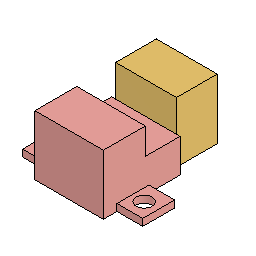
RoBo fan (Autodesk Fusion 360 archive; units mm, degrees)
design "male female connector"
Autodesk Fusion 360 part; units mm, degrees
sketch "Sketch1" plane through (0, 0, 0) normal (0, 0, 1) x (1, 0, 0) in component "male"
  line L0 (8.57, -9.6) -> (-8.57, -9.6)
  line L1 (-8.57, -9.6) -> (-8.57, 9.6)
  line L2 (-8.57, 9.6) -> (8.57, 9.6)
  line L3 (8.57, 9.6) -> (8.57, -9.6)
  line L4 (8.57, -9.6) -> (-8.57, 9.6) construction
  line L5 (-8.57, -9.6) -> (8.57, 9.6) construction
  line L6 (15.03, 1.8) -> (15.03, -6.2)
  line L7 (-15.03, -6.2) -> (-15.03, 1.8)
  line L8 (0, -6.2) -> (0, 0) construction
  circle A0 centre (-11.58, -2.4) radius 2
  circle A1 centre (11.58, -2.4) radius 2
  line L9 (-11.58, -2.4) -> (11.58, -2.4) construction
  line L10 (0, -2.4) -> (0, -6.2) construction
  line L11 (8.57, 0.9) -> (-8.57, 0.9)
  line L12 (-15.03, 1.8) -> (-8.57, 1.8)
  line L13 (8.57, 1.8) -> (15.03, 1.8)
  line L14 (15.03, -6.2) -> (8.57, -6.2)
  line L15 (-8.57, -6.2) -> (-15.03, -6.2)
  dimension "d1" = 17.14
  dimension "d2" = 19.2
  dimension "d4" = 8
  dimension "d5" = 7.8
  dimension "d6" = 4
  dimension "d7" = 23.16
  dimension "d8" = 3.8
  dimension "d9" = 6.46
  dimension "d14" = 8.7
  constraint horizontal L0
  constraint perpendicular L0 L1
  constraint parallel L0 L2
  constraint parallel L1 L3
  constraint coincident L4 L8.end
  constraint coincident L5 L8.end
  constraint coincident L8.end origin
  constraint horizontal L12
  constraint vertical L6
  constraint horizontal L14
  constraint vertical L7
  constraint vertical L8
  constraint coincident A0.centre L9.start
  constraint coincident A1.centre L9.end
  constraint horizontal L9
  constraint equal A0 A1
  constraint midpoint L9 L10.start
  constraint vertical L10
  constraint coincident L3 L11.start
  constraint coincident L1 L11.end
  constraint perpendicular L1 L11
  constraint coincident L3 L13.start
  constraint collinear L12 L13
  constraint coincident L1 L12.end
  constraint collinear L14 L15
  constraint coincident L3 L14.end
  constraint coincident L1 L15.start
  constraint equal L14 L15
  measures "d1" distance of L1.end L2.end
  measures "d2" distance of L0.end L1.end
  measures "d4" distance of L7.end L7.start
  measures "d5" distance of L1.end L12
  measures "d6" diameter of A0
  measures "d7" distance of A0.centre A1.centre
  measures "d8" distance of L9 L14
  measures "d9" distance of L1 L7.end
  measures "d14" distance of L2 L11
extrude "Extrude1" add sketch "Sketch1" along normal blind 1.74 contours L3 L6 L13 L14 | L1 L7 L12 L15 makes body 1 at (-11.7765, 1.0648, 0) makes body 2 at (11.7765, 1.0648, 0) in component "male"
extrude "Extrude3" add sketch "Sketch1" along normal blind 8.4 contours L1 L2 L3 L11 bodies 1 2 in component "male"
extrude "Extrude4" add sketch "Sketch1" along normal blind 15 contours L0 L1 L3 L11 bodies 1 in component "male"
sketch "Sketch1 (2)" plane through (0, 0, 0) normal (0, 0, 1) x (1, 0, 0) in component "female"
  line L0 (9.3617, 28.1045) -> (-5.8783, 28.1045)
  line L1 (-5.8783, 28.1045) -> (-5.8783, 47.0045)
  line L2 (-5.8783, 47.0045) -> (9.3617, 47.0045)
  line L3 (9.3617, 47.0045) -> (9.3617, 28.1045)
  line L4 (9.3617, 36.8045) -> (-5.8783, 36.8045)
  dimension "d19" = 15.24
  dimension "d20" = 18.9
  dimension "d21" = 8.7
  constraint horizontal L0
  constraint vertical L1
  constraint horizontal L2
  constraint vertical L3
  constraint coincident L3 L4.start
  constraint coincident L1 L4.end
  constraint perpendicular L1 L4
  measures "d19" distance of L0.start L0.end
  measures "d20" distance of L0.start L2.end
  measures "d21" distance of L0 L4
extrude "Extrude1'" add sketch "Sketch1 (2)" along normal blind 6 separate body contours L0 L1 L3 L4 makes body 3 in component "female"
extrude "Extrude2" add sketch "Sketch1 (2)" along normal blind 15.1 contours L1 L2 L3 L4 bodies 3 in component "female"
component "male" placed x (1, 0, 0) y (0, 1, 0) z (0, 0, 1) at (0, 0, 0)
component "female" placed x (1, 0, 0) y (0, 1, 0) z (0, 0, 1) at (-1.7417, -27.1365, 1.2)
equation "d1 = ( 5.08 * 3 ) * 1 mm + 1.9 mm"
equation "d7 = ( 5.08 * 2 ) * 1 mm + 13 mm"
equation "d19 = ( 5.08 * 3 ) * 1 mm"
